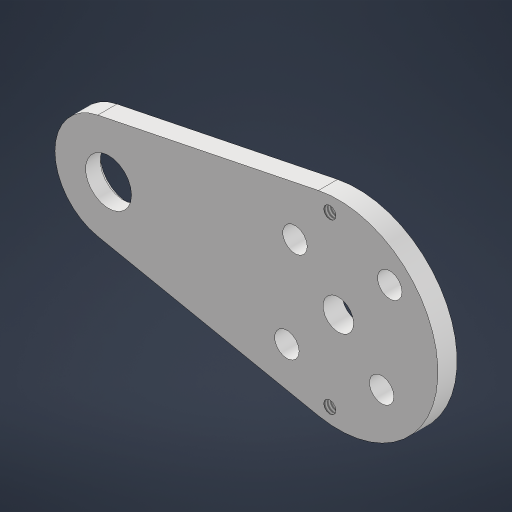
# Autodesk Inventor part: Dribler_main
Saved by Autodesk Inventor 2024.2 (Build 282272000, 272)
## iProperties
Created: 2023-12-22
Part Number: Dribler_main
Material: 一般
Document SubType Name: Modeling
Designer: Hanaoka
Density: 1 g/cm^3
Appearance: 既定
Author: Hanaoka
Autodesk Inventor part; units mm, degrees
ref_plane "YZ Plane" through (0, 0, 0) normal (1, 0, 0) x (0, 1, 0)
ref_plane "XZ Plane" through (0, 0, 0) normal (0, 1, 0) x (-1, 0, 0)
ref_plane "XY Plane" through (0, 0, 0) normal (0, 0, 1) x (1, 0, 0)
sketch "スケッチ1" plane through (0, 0, 0) normal (0, 0, 1) x (1, 0, 0)
  circle A0 centre (0, 0) radius 13
  line L0 (-2.6, 12.7373) -> (-31.4, 6.8586)
  line L1 (-2.6, -12.7373) -> (-31.4, -6.8586)
  arc A1 (-31.4, 6.8586) -> (-31.4, -6.8586) centre (-30, 0) ccw
  line L2 (-47, 0) -> (23, 0) projected
  circle A2 centre (-5.6569, 5.6569) radius 1.6 projected
  circle A3 centre (6.7175, 6.7175) radius 1.6 projected
  circle A4 centre (5.6569, -5.6569) radius 1.6 projected
  circle A5 centre (-6.7175, -6.7175) radius 1.6 projected
  circle A6 centre (0, 0) radius 2
  dimension "d0" = 30
  dimension "d1" = 26
  dimension "d2" = 7
  dimension "d5" = 4
  constraints: 4 end point, 4 point on circle, 4 tangent, 3 centre point, 2 coincident, 1 point on line
  measures "d0" distance of point (0, 0) A1.centre
  measures "d1" diameter of A0
  measures "d2" radius of A1
  measures "d5" diameter of A6
extrude "押し出し1" add sketch "スケッチ1" along normal blind 2.5 contours L2 A6 A0 | A0 L2 A6 | A0 L2 A1 L0 | L1 A1 L2 A0
sketch "スケッチ2" plane through (0, 0, 0) normal (0, 0, -1) x (-1, 0, 0)
  circle A0 centre (30, 0) radius 3
  circle A1 centre (30, 0) radius 1.5
  circle A2 centre (30, 0) radius 3.6
  line L0 (47, 0) -> (-23, 0) projected
  arc A3 (31.4, -6.8586) -> (31.4, 6.8586) centre (30, 0) ccw projected
  circle A4 centre (1.1112, 11) radius 0.8
  circle A5 centre (1.1112, -11) radius 0.8
  circle A6 centre (1.1112, 11) radius 2 construction
  circle A7 centre (1.1112, -11) radius 2 construction
  line L1 (2.6, 12.7373) -> (31.4, 6.8586) projected
  circle A8 centre (5.6569, 5.6569) radius 1.6 projected
  circle A9 centre (5.6569, 5.6569) radius 1.6
  circle A10 centre (6.7175, -6.7175) radius 1.6
  circle A11 centre (5.6569, 5.6569) radius 3 construction
  circle A12 centre (6.7175, -6.7175) radius 3 construction
  point P0 (0, 0)
  dimension "d6" = 6
  dimension "d7" = 3
  dimension "d8" = 7.2
  dimension "d13" = 1.6
  dimension "d15" = 4
  dimension "d16" = 6
  dimension "d18" = 22
  constraints: 11 centre point, 7 coincident, 3 equal radius, 1 point on line, 1 tangent, 1 vertical alignment, 5 other
  measures "d6" diameter of A0
  measures "d7" diameter of A1
  measures "d8" diameter of A2
  measures "d13" diameter of A4
  measures "d15" diameter of A7
  measures "d16" diameter of A12
  measures "d18" distance of A5.centre A6.centre
extrude "押し出し2" cut sketch "スケッチ2" against normal blind 0.6 contours L0 A1 A0 | L0 A2 A0 | A0 L0 A2 | A0 L0 A1 | L0 A1 | A1 L0
extrude "押し出し3" cut sketch "スケッチ2" against normal up to surface (2.5 mm away) contours L0 A1 A0 | A0 L0 A1 | L0 A1 | A1 L0 | A4 | A5
thread "ねじ1" size "M2x0.4" class "6H" standard "ANSI Metric M Profile" full length
thread "ねじ2" size "M2x0.4" class "6H" standard "ANSI Metric M Profile" full length
